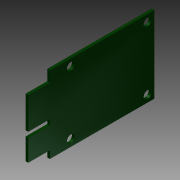
# Autodesk Inventor part: HidhSpeedIOShield01
Saved by Autodesk Inventor 2013 (Build 170138000, 138)
## iProperties
Created: 2014-07-14
Part Number: HidhSpeedIOShield01
Material: PCB(1)
Document SubType Name: Modeling
Designer: spichelh
Density: 1 g/cm^3
Author: spichelh
Autodesk Inventor part; units mm, degrees
ref_plane "YZ Plane" through (0, 0, 0) normal (1, 0, 0) x (0, 1, 0)
ref_plane "XZ Plane" through (0, 0, 0) normal (0, 1, 0) x (-1, 0, 0)
ref_plane "XY Plane" through (0, 0, 0) normal (0, 0, 1) x (1, 0, 0)
sketch "Sketch1" plane through (0, 0, 0) normal (1, 0, 0) x (0, 1, 0)
  line L0 (0, 0) -> (27.94, 0)
  line L1 (27.94, 0) -> (27.94, 38.1)
  line L2 (13.97, 0) -> (13.97, 11.6982) construction
  circle A0 centre (2.54, 2.54) radius 1.4
  circle A1 centre (25.4, 2.54) radius 1.4
  line L3 (0, 38.1) -> (2.74, 38.1)
  line L4 (2.74, 38.1) -> (2.74, 46)
  line L5 (2.74, 46) -> (10.54, 46)
  line L6 (10.54, 46) -> (10.54, 38.1)
  line L7 (10.54, 38.1) -> (12.54, 38.1)
  line L8 (12.54, 38.1) -> (12.54, 46)
  line L9 (12.54, 46) -> (24.04, 46)
  line L10 (24.04, 46) -> (24.04, 38.1)
  line L11 (24.04, 38.1) -> (27.94, 38.1)
  line L12 (0, 0) -> (0, 38.1)
  circle A2 centre (2.54, 30.48) radius 1.397
  circle A3 centre (25.4, 30.48) radius 1.397
  point P0 (13.97, 5.8491)
  dimension "d0" = 27.94
  dimension "d5" = 2.8
  dimension "d6" = 2.54
  dimension "d21" = 7.8
  dimension "d23" = 2
  dimension "d24" = 11.5
  dimension "d27" = 38.1
  dimension "d29" = 3.9
  dimension "d30" = 7.9
  dimension "d31" = 2.54
  dimension "d32" = 2.794
  dimension "d33" = 2.54
  dimension "d34" = 7.62
  constraints: 27 end point, 4 centre point, 3 collinear, 2 midpoint, 2 perpendicular, 2 symmetric about line, 2 vertical, 1 horizontal, 1 parallel, 2 other
  measures "d0" distance of L0.start L0.end
  measures "d5" diameter of A0
  measures "d6" distance from line of L0 A0.centre
  measures "d21" distance between parallel lines of L6 L4
  measures "d23" distance between parallel lines of L6 L8
  measures "d24" distance between parallel lines of L8 L10
  measures "d27" distance of L1.end L0.end
  measures "d29" distance between parallel lines of L10 L1
  measures "d30" distance between parallel lines of L3 L5
  measures "d31" distance from line of L12 A0.centre
  measures "d32" diameter of A2
  measures "d33" distance from line of L12 A2.centre
  measures "d34" distance from line of L3 A2.centre
extrude "Extrusion1" add sketch "Sketch1" along normal blind 1
body "Solid1"
